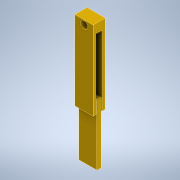
# Autodesk Inventor part: pendel
Saved by Autodesk Inventor 2021 (Build 250183000, 183)
## iProperties
Created: 2021-02-09
Part Number: pendel
Material: Generic
Document SubType Name: Modeling
Designer: Emil
Density: 1 g/cm^3
Appearance: Gold
Author: Emil
Autodesk Inventor part; units mm, degrees
ref_plane "YZ Plane" through (0, 0, 0) normal (1, 0, 0) x (0, 1, 0)
ref_plane "XZ Plane" through (0, 0, 0) normal (0, 1, 0) x (-1, 0, 0)
ref_plane "XY Plane" through (0, 0, 0) normal (0, 0, 1) x (1, 0, 0)
sketch "Sketch1" plane through (0, 0, 0) normal (0, 0, 1) x (1, 0, 0)
  point P0 (0, 0)
sketch "Sketch2" plane through (0, 0, 0) normal (0, 0, 1) x (1, 0, 0)
  line L0 (-15, 130) -> (15, 130)
  line L1 (15, 130) -> (15, 0)
  line L2 (15, 0) -> (-15, 0)
  line L3 (-15, 0) -> (-15, 130)
  point P0 (0, 0)
  point P1 (0, 0)
  dimension "d0" = 30
  dimension "d1" = 130
  constraints: 8 end point, 2 parallel, 1 coincident, 1 horizontal, 1 midpoint, 1 perpendicular
  measures "d0" distance of L0.start L0.end
  measures "d1" distance of L0.end L1.end
extrude "Extrusion1" add sketch "Sketch2" along normal blind 5
ref_plane "Work Plane1" through (0, 0, -10) normal (0, 0, -1) x (-1, 0, 0)
sketch "Sketch4" plane through (0, 0, -10) normal (0, 0, -1) x (-1, 0, 0)
  line L0 (-15, 0) -> (-15, 130) projected
  line L1 (15, 0) -> (-15, 0) projected
  line L2 (-15, 130) -> (15, 130)
  line L3 (15, 130) -> (15, 0)
  line L4 (15, 0) -> (-15, 0)
  line L5 (-15, 0) -> (-15, 130)
  point P0 (0, 0)
  constraints: 8 end point, 2 parallel, 1 horizontal, 1 perpendicular
extrude "Extrusion3" add sketch "Sketch4" along normal blind 5
sketch "Sketch5" plane through (0, 0, -10) normal (0, 0, 1) x (1, 0, 0)
  line L0 (-15, 130) -> (-15, 0) projected
  line L1 (15, 130) -> (15, 0) projected
  line L2 (-15, 130) -> (15, 130)
  line L3 (15, 130) -> (15, 115)
  line L4 (15, 115) -> (-15, 115)
  line L5 (-15, 115) -> (-15, 130)
  point P0 (0, 0)
  point P1 (15, 130)
  dimension "d12" = 15
  constraints: 8 end point, 2 parallel, 1 horizontal, 1 perpendicular, 1 point on line
  measures "d12" distance between parallel lines of L4 L2
extrude "Extrusion4" add sketch "Sketch5" along normal blind 10
sketch "Sketch6" plane through (0, 0, -10) normal (0, 0, 1) x (1, 0, 0)
  circle A0 centre (0, 10) radius 2.5
  line L0 (-15, 0) -> (15, 0) projected
  point P0 (0, 0)
  dimension "d15" = 5
  dimension "d16" = 10
  dimension "d45" = 18.0278
  constraints: 1 centre point
  measures "d15" diameter of A0
  measures "d16" distance from line of L0 A0.centre
  measures "d45" distance of L0.end A0.centre
extrude "Extrusion5" add sketch "Sketch6" along normal blind 10
ref_plane "Work Plane2" through (0, 0, -5) normal (0, 0, 1) x (1, 0, 0)
sketch "Sketch7" plane through (0, 0, -5) normal (0, 0, 1) x (1, 0, 0)
  line L0 (-15, 0) -> (-15, 115) projected
  line L1 (-15, 20) -> (15, 20)
  line L2 (15, 20) -> (15, -80)
  line L3 (15, -80) -> (-15, -80)
  line L4 (-15, -80) -> (-15, 20)
  line L5 (15, 0) -> (-15, 0) projected
  circle A0 centre (0, 10) radius 2.5 projected
  circle A1 centre (0, 10) radius 4
  point P0 (0, 0)
  dimension "d20" = 30
  dimension "d21" = 100
  dimension "d22" = 20
  dimension "d23" = 8
  constraints: 8 end point, 2 parallel, 1 centre point, 1 coincident, 1 horizontal, 1 perpendicular, 1 point on line
  measures "d20" distance between parallel lines of L4 L2
  measures "d21" distance of L1.end L2.end
  measures "d22" distance between parallel lines of L5 L1
  measures "d23" diameter of A1
extrude "Extrusion6" add sketch "Sketch7" along normal mid plane 7 contours L5 L2 L3 L4 | L0 L1 L2 L5
sketch "Sketch9" plane through (0, 0, 5) normal (0, 0, 1) x (1, 0, 0)
  line L0 (15, 130) -> (-15, 130) projected
  line L1 (15, 0) -> (15, 130) projected
  line L2 (0, 84.3715) -> (0, -83.7026)
  line L3 (-15, 0) -> (15, 0) projected
  line L4 (-15, 122.5) -> (15, 122.5)
  line L5 (-15, 115) -> (15, 115) projected
  circle A0 centre (0, 122.5) radius 6
  point P0 (0, 0)
  point P1 (0, 0)
  dimension "d41" = 7.5
  dimension "d42" = 12
  dimension "d46" = 15
  dimension "d47" = 45.6285
  dimension "d48" = 213.7026
  constraints: 4 end point, 2 midpoint, 2 point on line, 1 centre point, 1 perpendicular, 1 vertical
  measures "d41" distance between parallel lines of L5 L4
  measures "d42" diameter of A0
  measures "d46" distance from line of A0.centre L1
  measures "d47" distance from line of L2.start L0
  measures "d48" distance from line of L2.end L0
sketch "Sketch10" plane through (0, 0, -1.5) normal (0, 0, 1) x (1, 0, 0)
  point P0 (0, 0)
sketch "Sketch11" plane through (-15, -80, -1.5) normal (-1, 0, 0) x (0, 0, 1)
  line L0 (-5.6394, 0.8654) -> (-5.6394, 102.3274) construction
  line L1 (-5.6394, 102.3274) -> (-2.3913, 102.3274) construction
  line L2 (-2.3913, 102.3274) -> (-2.3913, 0.8654) construction
  line L3 (-2.3913, 0.8654) -> (-5.6394, 0.8654) construction
  line L4 (-5.6394, 1.7568) -> (-4.0835, 1.6401)
  line L5 (-4.0835, 1.6401) -> (-4.0835, 1.2868)
  line L6 (-4.0835, 1.2868) -> (-5.6394, 1.1701)
  line L7 (-5.6394, 1.1701) -> (-5.6394, 1.7568)
  line L8 (-5.6394, 2.7681) -> (-4.0835, 2.6514)
  line L9 (-4.0835, 2.6514) -> (-4.0835, 2.2981)
  line L10 (-4.0835, 2.2981) -> (-5.6394, 2.1814)
  line L11 (-5.6394, 2.1814) -> (-5.6394, 2.7681)
  line L12 (-1.4611, 4.8719) -> (-1.4611, 3.3224)
  line L13 (-1.4611, 3.3224) -> (-1.8695, 3.3224)
  line L14 (-1.8695, 3.3224) -> (-1.8695, 3.8313)
  line L15 (-1.8695, 3.8313) -> (-5.0527, 3.8313)
  line L16 (-5.0527, 3.8313) -> (-5.0527, 3.3224)
  line L17 (-5.0527, 3.3224) -> (-5.4611, 3.3224)
  line L18 (-5.4611, 3.3224) -> (-5.4611, 4.8719)
  line L19 (-5.4611, 4.8719) -> (-5.0527, 4.8719)
  line L20 (-5.0527, 4.8719) -> (-5.0527, 4.3629)
  line L21 (-5.0527, 4.3629) -> (-1.8695, 4.3629)
  line L22 (-1.8695, 4.3629) -> (-1.8695, 4.8719)
  line L23 (-1.8695, 4.8719) -> (-1.4611, 4.8719)
  spline S0 degree 2 poles (-1.4028, 8.1166) (-1.4028, 7.7049) (-1.8728, 7.2414) (-2.3817, 7.2414) knots 0 0 0 1 2 2 2
  line L24 (-2.3817, 7.2414) -> (-4.0446, 7.2414)
  line L25 (-4.0446, 7.2414) -> (-4.0446, 6.901)
  line L26 (-4.0446, 6.901) -> (-4.4627, 6.901)
  line L27 (-4.4627, 6.901) -> (-4.4627, 7.2414)
  line L28 (-4.4627, 7.2414) -> (-5.325, 7.2414)
  line L29 (-5.325, 7.2414) -> (-5.325, 7.7471)
  line L30 (-5.325, 7.7471) -> (-4.4627, 7.7471)
  line L31 (-4.4627, 7.7471) -> (-4.4627, 8.6774)
  line L32 (-4.4627, 8.6774) -> (-4.0446, 8.6774)
  line L33 (-4.0446, 8.6774) -> (-4.0446, 7.7471)
  line L34 (-4.0446, 7.7471) -> (-2.6151, 7.7471)
  spline S1 degree 2 poles (-2.6151, 7.7471) (-2.3882, 7.7471) (-2.1386, 7.7633) (-2.0316, 7.8184) knots 0 0 0 1 2 2 2
  spline S2 degree 2 poles (-2.0316, 7.8184) (-1.9376, 7.8638) (-1.8436, 8.068) (-1.8436, 8.243) knots 0 0 0 1 2 2 2
  spline S3 degree 2 poles (-1.8436, 8.243) (-1.8436, 8.3662) (-1.9182, 8.5963) (-1.9408, 8.6482) knots 0 0 0 1 2 2 2
  line L35 (-1.9408, 8.6482) -> (-1.9408, 8.6774)
  line L36 (-1.9408, 8.6774) -> (-1.487, 8.6774)
  spline S4 degree 2 poles (-1.487, 8.6774) (-1.4481, 8.5347) (-1.4028, 8.243) (-1.4028, 8.1166) knots 0 0 0 1 2 2 2
  line L37 (-1.4611, 11.4067) -> (-1.4611, 10.901)
  line L38 (-1.4611, 10.901) -> (-3.1726, 10.901)
  spline S5 degree 2 poles (-3.1726, 10.901) (-3.3801, 10.901) (-3.7366, 10.8621) (-3.8436, 10.8038) knots 0 0 0 1 2 2 2
  spline S6 degree 2 poles (-3.8436, 10.8038) (-3.957, 10.7422) (-4.0673, 10.5218) (-4.0673, 10.3338) knots 0 0 0 1 2 2 2
  spline S7 degree 2 poles (-4.0673, 10.3338) (-4.0673, 10.1458) (-3.8663, 9.7471) (-3.7042, 9.5558) knots 0 0 0 1 2 2 2
  line L39 (-3.7042, 9.5558) -> (-1.4611, 9.5558)
  line L40 (-1.4611, 9.5558) -> (-1.4611, 9.0501)
  line L41 (-1.4611, 9.0501) -> (-5.6394, 9.0501)
  line L42 (-5.6394, 9.0501) -> (-5.6394, 9.5558)
  line L43 (-5.6394, 9.5558) -> (-4.1288, 9.5558)
  spline S8 degree 2 poles (-4.1288, 9.5558) (-4.3331, 9.7827) (-4.547, 10.2203) (-4.547, 10.4667) knots 0 0 0 1 2 2 2
  spline S9 degree 2 poles (-4.547, 10.4667) (-4.547, 10.9075) (-3.9635, 11.4067) (-3.4092, 11.4067) knots 0 0 0 1 2 2 2
  line L44 (-3.4092, 11.4067) -> (-1.4611, 11.4067)
  line L45 (-3.9214, 13.7082) -> (-3.9214, 13.6822)
  spline S10 degree 2 poles (-3.9214, 13.6822) (-3.9376, 13.6239) (-3.9441, 13.4975) (-3.9441, 13.4099) knots 0 0 0 1 2 2 2
  spline S11 degree 2 poles (-3.9441, 13.4099) (-3.9441, 13.2057) (-3.7658, 12.8038) (-3.5908, 12.6223) knots 0 0 0 1 2 2 2
  line L46 (-3.5908, 12.6223) -> (-1.4611, 12.6223)
  line L47 (-1.4611, 12.6223) -> (-1.4611, 12.1166)
  line L48 (-1.4611, 12.1166) -> (-4.4627, 12.1166)
  line L49 (-4.4627, 12.1166) -> (-4.4627, 12.6223)
  line L50 (-4.4627, 12.6223) -> (-4.0154, 12.6223)
  spline S12 degree 2 poles (-4.0154, 12.6223) (-4.2618, 12.8978) (-4.4627, 13.3095) (-4.4627, 13.5039) knots 0 0 0 1 2 2 2
  spline S13 degree 2 poles (-4.4627, 13.5039) (-4.4627, 13.5817) (-4.4562, 13.6595) (-4.4465, 13.7082) knots 0 0 0 1 2 2 2
  line L51 (-4.4465, 13.7082) -> (-3.9214, 13.7082)
  line L52 (-1.4611, 14.6158) -> (-1.4611, 14.1101)
  line L53 (-1.4611, 14.1101) -> (-4.4627, 14.1101)
  line L54 (-4.4627, 14.1101) -> (-4.4627, 14.6158)
  line L55 (-4.4627, 14.6158) -> (-1.4611, 14.6158)
  line L56 (-4.9619, 14.6514) -> (-4.9619, 14.0777)
  line L57 (-4.9619, 14.0777) -> (-5.487, 14.0777)
  line L58 (-5.487, 14.0777) -> (-5.487, 14.6514)
  line L59 (-5.487, 14.6514) -> (-4.9619, 14.6514)
  line L60 (-4.4627, 17.7146) -> (-1.4611, 16.5834)
  line L61 (-1.4611, 16.5834) -> (-1.4611, 16.1296)
  line L62 (-1.4611, 16.1296) -> (-4.4627, 15.008)
  line L63 (-4.4627, 15.008) -> (-4.4627, 15.5558)
  line L64 (-4.4627, 15.5558) -> (-2.1515, 16.3759)
  line L65 (-2.1515, 16.3759) -> (-4.4627, 17.1895)
  line L66 (-4.4627, 17.1895) -> (-4.4627, 17.7146)
  spline S14 degree 2 poles (-1.393, 19.4002) (-1.393, 18.6806) (-2.2002, 17.8897) (-2.9457, 17.8897) knots 0 0 0 1 2 2 2
  spline S15 degree 2 poles (-2.9457, 17.8897) (-3.6783, 17.8897) (-4.547, 18.6579) (-4.547, 19.277) knots 0 0 0 1 2 2 2
  spline S16 degree 2 poles (-4.547, 19.277) (-4.547, 19.5558) (-4.3849, 19.9869) (-4.2131, 20.1458) knots 0 0 0 1 2 2 2
  spline S17 degree 2 poles (-4.2131, 20.1458) (-4.0413, 20.3078) (-3.5454, 20.4796) (-3.1856, 20.4796) knots 0 0 0 1 2 2 2
  line L67 (-3.1856, 20.4796) -> (-2.91, 20.4796)
  line L68 (-2.91, 20.4796) -> (-2.91, 18.4018)
  spline S18 degree 2 poles (-2.91, 18.4018) (-2.3882, 18.4018) (-1.8339, 18.927) (-1.8339, 19.3937) knots 0 0 0 1 2 2 2
  spline S19 degree 2 poles (-1.8339, 19.3937) (-1.8339, 19.5591) (-1.9084, 19.88) (-1.9668, 20.0096) knots 0 0 0 1 2 2 2
  spline S20 degree 2 poles (-1.9668, 20.0096) (-2.0316, 20.1458) (-2.1451, 20.3338) (-2.1969, 20.3954) knots 0 0 0 1 2 2 2
  line L69 (-2.1969, 20.3954) -> (-2.1969, 20.4245)
  line L70 (-2.1969, 20.4245) -> (-1.6459, 20.4245)
  spline S21 degree 2 poles (-1.6459, 20.4245) (-1.6102, 20.337) (-1.5065, 20.0712) (-1.4773, 19.9675) knots 0 0 0 1 2 2 2
  spline S22 degree 2 poles (-1.4773, 19.9675) (-1.4352, 19.8216) (-1.393, 19.5817) (-1.393, 19.4002) knots 0 0 0 1 2 2 2
  spline S23 degree 2 poles (-3.2958, 19.9869) (-3.5, 19.9804) (-3.7982, 19.8962) (-3.8987, 19.8151) knots 0 0 0 1 2 2 2
  spline S24 degree 2 poles (-3.8987, 19.8151) (-4.0122, 19.7276) (-4.1321, 19.4521) (-4.1321, 19.2479) knots 0 0 0 1 2 2 2
  spline S25 degree 2 poles (-4.1321, 19.2479) (-4.1321, 19.0469) (-4.0122, 18.7649) (-3.8955, 18.6482) knots 0 0 0 1 2 2 2
  spline S26 degree 2 poles (-3.8955, 18.6482) (-3.7755, 18.5347) (-3.487, 18.418) (-3.2958, 18.4018) knots 0 0 0 1 2 2 2
  line L71 (-3.2958, 18.4018) -> (-3.2958, 19.9869)
  line L72 (-1.4611, 23.2252) -> (-1.4611, 22.7195)
  line L73 (-1.4611, 22.7195) -> (-4.4627, 22.7195)
  line L74 (-4.4627, 22.7195) -> (-4.4627, 23.2252)
  line L75 (-4.4627, 23.2252) -> (-1.4611, 23.2252)
  line L76 (-4.9619, 23.2608) -> (-4.9619, 22.6871)
  line L77 (-4.9619, 22.6871) -> (-5.487, 22.6871)
  line L78 (-5.487, 22.6871) -> (-5.487, 23.2608)
  line L79 (-5.487, 23.2608) -> (-4.9619, 23.2608)
  line L80 (-1.4611, 26.324) -> (-1.4611, 25.8184)
  line L81 (-1.4611, 25.8184) -> (-3.1726, 25.8184)
  spline S27 degree 2 poles (-3.1726, 25.8184) (-3.3801, 25.8184) (-3.7366, 25.7795) (-3.8436, 25.7211) knots 0 0 0 1 2 2 2
  spline S28 degree 2 poles (-3.8436, 25.7211) (-3.957, 25.6595) (-4.0673, 25.4391) (-4.0673, 25.2511) knots 0 0 0 1 2 2 2
  spline S29 degree 2 poles (-4.0673, 25.2511) (-4.0673, 25.0631) (-3.8663, 24.6644) (-3.7042, 24.4732) knots 0 0 0 1 2 2 2
  line L82 (-3.7042, 24.4732) -> (-1.4611, 24.4732)
  line L83 (-1.4611, 24.4732) -> (-1.4611, 23.9675)
  line L84 (-1.4611, 23.9675) -> (-4.4627, 23.9675)
  line L85 (-4.4627, 23.9675) -> (-4.4627, 24.4732)
  line L86 (-4.4627, 24.4732) -> (-4.1288, 24.4732)
  spline S30 degree 2 poles (-4.1288, 24.4732) (-4.3331, 24.7001) (-4.547, 25.1377) (-4.547, 25.384) knots 0 0 0 1 2 2 2
  spline S31 degree 2 poles (-4.547, 25.384) (-4.547, 25.8249) (-3.9635, 26.324) (-3.4092, 26.324) knots 0 0 0 1 2 2 2
  line L87 (-3.4092, 26.324) -> (-1.4611, 26.324)
  spline S32 degree 2 poles (-1.3898, 29.5623) (-1.3898, 29.2608) (-1.5519, 28.739) (-1.6426, 28.5672) knots 0 0 0 1 2 2 2
  line L88 (-1.6426, 28.5672) -> (-2.2099, 28.5672)
  line L89 (-2.2099, 28.5672) -> (-2.2099, 28.5931)
  spline S33 degree 2 poles (-2.2099, 28.5931) (-2.158, 28.6579) (-2.0348, 28.833) (-1.9668, 28.9788) knots 0 0 0 1 2 2 2
  spline S34 degree 2 poles (-1.9668, 28.9788) (-1.9052, 29.1052) (-1.8144, 29.4164) (-1.8144, 29.5817) knots 0 0 0 1 2 2 2
  spline S35 degree 2 poles (-1.8144, 29.5817) (-1.8144, 29.7017) (-1.8695, 29.9772) (-1.9149, 30.042) knots 0 0 0 1 2 2 2
  spline S36 degree 2 poles (-1.9149, 30.042) (-1.9765, 30.136) (-2.1159, 30.2203) (-2.2585, 30.2203) knots 0 0 0 1 2 2 2
  spline S37 degree 2 poles (-2.2585, 30.2203) (-2.4368, 30.2203) (-2.6216, 30.0258) (-2.6831, 29.7762) knots 0 0 0 1 2 2 2
  spline S38 degree 2 poles (-2.6831, 29.7762) (-2.7058, 29.679) (-2.7707, 29.3678) (-2.8063, 29.2349) knots 0 0 0 1 2 2 2
  spline S39 degree 2 poles (-2.8063, 29.2349) (-2.9068, 28.8913) (-3.3217, 28.5801) (-3.6167, 28.5801) knots 0 0 0 1 2 2 2
  spline S40 degree 2 poles (-3.6167, 28.5801) (-4.0251, 28.5801) (-4.534, 29.1928) (-4.534, 29.6984) knots 0 0 0 1 2 2 2
  spline S41 degree 2 poles (-4.534, 29.6984) (-4.534, 29.948) (-4.4109, 30.4537) (-4.3169, 30.6255) knots 0 0 0 1 2 2 2
  line L90 (-4.3169, 30.6255) -> (-3.7755, 30.6255)
  line L91 (-3.7755, 30.6255) -> (-3.7755, 30.5996)
  spline S42 degree 2 poles (-3.7755, 30.5996) (-3.9311, 30.4051) (-4.1094, 29.9318) (-4.1094, 29.6887) knots 0 0 0 1 2 2 2
  spline S43 degree 2 poles (-4.1094, 29.6887) (-4.1094, 29.4391) (-3.8987, 29.0955) (-3.688, 29.0955) knots 0 0 0 1 2 2 2
  spline S44 degree 2 poles (-3.688, 29.0955) (-3.4968, 29.0955) (-3.312, 29.2997) (-3.2536, 29.5266) knots 0 0 0 1 2 2 2
  spline S45 degree 2 poles (-3.2536, 29.5266) (-3.2245, 29.6368) (-3.1661, 29.9156) (-3.1305, 30.068) knots 0 0 0 1 2 2 2
  spline S46 degree 2 poles (-3.1305, 30.068) (-3.0462, 30.3986) (-2.6605, 30.7357) (-2.3266, 30.7357) knots 0 0 0 1 2 2 2
  spline S47 degree 2 poles (-2.3266, 30.7357) (-2.1321, 30.7357) (-1.7885, 30.5834) (-1.6621, 30.4343) knots 0 0 0 1 2 2 2
  spline S48 degree 2 poles (-1.6621, 30.4343) (-1.5292, 30.2754) (-1.3898, 29.8702) (-1.3898, 29.5623) knots 0 0 0 1 2 2 2
  spline S49 degree 2 poles (-1.4028, 32.1133) (-1.4028, 31.7017) (-1.8728, 31.2381) (-2.3817, 31.2381) knots 0 0 0 1 2 2 2
  line L92 (-2.3817, 31.2381) -> (-4.0446, 31.2381)
  line L93 (-4.0446, 31.2381) -> (-4.0446, 30.8978)
  line L94 (-4.0446, 30.8978) -> (-4.4627, 30.8978)
  line L95 (-4.4627, 30.8978) -> (-4.4627, 31.2381)
  line L96 (-4.4627, 31.2381) -> (-5.325, 31.2381)
  line L97 (-5.325, 31.2381) -> (-5.325, 31.7438)
  line L98 (-5.325, 31.7438) -> (-4.4627, 31.7438)
  line L99 (-4.4627, 31.7438) -> (-4.4627, 32.6741)
  line L100 (-4.4627, 32.6741) -> (-4.0446, 32.6741)
  line L101 (-4.0446, 32.6741) -> (-4.0446, 31.7438)
  line L102 (-4.0446, 31.7438) -> (-2.6151, 31.7438)
  spline S50 degree 2 poles (-2.6151, 31.7438) (-2.3882, 31.7438) (-2.1386, 31.76) (-2.0316, 31.8151) knots 0 0 0 1 2 2 2
  spline S51 degree 2 poles (-2.0316, 31.8151) (-1.9376, 31.8605) (-1.8436, 32.0647) (-1.8436, 32.2398) knots 0 0 0 1 2 2 2
  spline S52 degree 2 poles (-1.8436, 32.2398) (-1.8436, 32.3629) (-1.9182, 32.5931) (-1.9408, 32.645) knots 0 0 0 1 2 2 2
  line L103 (-1.9408, 32.645) -> (-1.9408, 32.6741)
  line L104 (-1.9408, 32.6741) -> (-1.487, 32.6741)
  spline S53 degree 2 poles (-1.487, 32.6741) (-1.4481, 32.5315) (-1.4028, 32.2398) (-1.4028, 32.1133) knots 0 0 0 1 2 2 2
  line L105 (-3.9214, 34.6385) -> (-3.9214, 34.6125)
  spline S54 degree 2 poles (-3.9214, 34.6125) (-3.9376, 34.5542) (-3.9441, 34.4278) (-3.9441, 34.3403) knots 0 0 0 1 2 2 2
  spline S55 degree 2 poles (-3.9441, 34.3403) (-3.9441, 34.136) (-3.7658, 33.7341) (-3.5908, 33.5526) knots 0 0 0 1 2 2 2
  line L106 (-3.5908, 33.5526) -> (-1.4611, 33.5526)
  line L107 (-1.4611, 33.5526) -> (-1.4611, 33.0469)
  line L108 (-1.4611, 33.0469) -> (-4.4627, 33.0469)
  line L109 (-4.4627, 33.0469) -> (-4.4627, 33.5526)
  line L110 (-4.4627, 33.5526) -> (-4.0154, 33.5526)
  spline S56 degree 2 poles (-4.0154, 33.5526) (-4.2618, 33.8281) (-4.4627, 34.2398) (-4.4627, 34.4343) knots 0 0 0 1 2 2 2
  spline S57 degree 2 poles (-4.4627, 34.4343) (-4.4627, 34.5121) (-4.4562, 34.5898) (-4.4465, 34.6385) knots 0 0 0 1 2 2 2
  line L111 (-4.4465, 34.6385) -> (-3.9214, 34.6385)
  line L112 (-1.4611, 37.3646) -> (-1.4611, 36.8589)
  line L113 (-1.4611, 36.8589) -> (-1.7917, 36.8589)
  spline S58 degree 2 poles (-1.7917, 36.8589) (-1.5875, 36.6255) (-1.3768, 36.2074) (-1.3768, 35.948) knots 0 0 0 1 2 2 2
  spline S59 degree 2 poles (-1.3768, 35.948) (-1.3768, 35.7535) (-1.5065, 35.4067) (-1.6459, 35.2803) knots 0 0 0 1 2 2 2
  spline S60 degree 2 poles (-1.6459, 35.2803) (-1.7853, 35.1506) (-2.2099, 35.008) (-2.5146, 35.008) knots 0 0 0 1 2 2 2
  line L114 (-2.5146, 35.008) -> (-4.4627, 35.008)
  line L115 (-4.4627, 35.008) -> (-4.4627, 35.5137)
  line L116 (-4.4627, 35.5137) -> (-2.7512, 35.5137)
  spline S61 degree 2 poles (-2.7512, 35.5137) (-2.5113, 35.5137) (-2.1969, 35.5493) (-2.0802, 35.6109) knots 0 0 0 1 2 2 2
  spline S62 degree 2 poles (-2.0802, 35.6109) (-1.9635, 35.6725) (-1.8566, 35.8832) (-1.8566, 36.0809) knots 0 0 0 1 2 2 2
  spline S63 degree 2 poles (-1.8566, 36.0809) (-1.8566, 36.2657) (-2.0673, 36.6839) (-2.2196, 36.8589) knots 0 0 0 1 2 2 2
  line L117 (-2.2196, 36.8589) -> (-4.4627, 36.8589)
  line L118 (-4.4627, 36.8589) -> (-4.4627, 37.3646)
  line L119 (-4.4627, 37.3646) -> (-1.4611, 37.3646)
  spline S64 degree 2 poles (-1.393, 39.29) (-1.393, 38.9788) (-1.5843, 38.4634) (-1.7788, 38.2787) knots 0 0 0 1 2 2 2
  spline S65 degree 2 poles (-1.7788, 38.2787) (-1.97, 38.0939) (-2.56, 37.8897) (-2.9554, 37.8897) knots 0 0 0 1 2 2 2
  spline S66 degree 2 poles (-2.9554, 37.8897) (-3.3509, 37.8897) (-3.9279, 38.1004) (-4.1224, 38.2787) knots 0 0 0 1 2 2 2
  spline S67 degree 2 poles (-4.1224, 38.2787) (-4.3201, 38.4569) (-4.5308, 38.9853) (-4.5308, 39.29) knots 0 0 0 1 2 2 2
  spline S68 degree 2 poles (-4.5308, 39.29) (-4.5308, 39.5364) (-4.3914, 39.9967) (-4.3006, 40.1749) knots 0 0 0 1 2 2 2
  line L120 (-4.3006, 40.1749) -> (-3.7334, 40.1749)
  line L121 (-3.7334, 40.1749) -> (-3.7334, 40.1458)
  spline S69 degree 2 poles (-3.7334, 40.1458) (-3.7788, 40.0907) (-3.8955, 39.9221) (-3.957, 39.8022) knots 0 0 0 1 2 2 2
  spline S70 degree 2 poles (-3.957, 39.8022) (-4.0089, 39.6952) (-4.09, 39.4099) (-4.09, 39.2803) knots 0 0 0 1 2 2 2
  spline S71 degree 2 poles (-4.09, 39.2803) (-4.09, 38.8881) (-3.4968, 38.4116) (-2.9554, 38.4116) knots 0 0 0 1 2 2 2
  spline S72 degree 2 poles (-2.9554, 38.4116) (-2.4271, 38.4116) (-1.8339, 38.8719) (-1.8339, 39.2803) knots 0 0 0 1 2 2 2
  spline S73 degree 2 poles (-1.8339, 39.2803) (-1.8339, 39.5266) (-2.0381, 39.974) (-2.1969, 40.1458) knots 0 0 0 1 2 2 2
  line L122 (-2.1969, 40.1458) -> (-2.1969, 40.1749)
  line L123 (-2.1969, 40.1749) -> (-1.6297, 40.1749)
  spline S74 degree 2 poles (-1.6297, 40.1749) (-1.594, 40.1004) (-1.4935, 39.8735) (-1.4708, 39.7827) knots 0 0 0 1 2 2 2
  spline S75 degree 2 poles (-1.4708, 39.7827) (-1.4319, 39.6531) (-1.393, 39.4488) (-1.393, 39.29) knots 0 0 0 1 2 2 2
  spline S76 degree 2 poles (-1.4028, 41.5428) (-1.4028, 41.1312) (-1.8728, 40.6676) (-2.3817, 40.6676) knots 0 0 0 1 2 2 2
  line L124 (-2.3817, 40.6676) -> (-4.0446, 40.6676)
  line L125 (-4.0446, 40.6676) -> (-4.0446, 40.3273)
  line L126 (-4.0446, 40.3273) -> (-4.4627, 40.3273)
  line L127 (-4.4627, 40.3273) -> (-4.4627, 40.6676)
  line L128 (-4.4627, 40.6676) -> (-5.325, 40.6676)
  line L129 (-5.325, 40.6676) -> (-5.325, 41.1733)
  line L130 (-5.325, 41.1733) -> (-4.4627, 41.1733)
  line L131 (-4.4627, 41.1733) -> (-4.4627, 42.1036)
  line L132 (-4.4627, 42.1036) -> (-4.0446, 42.1036)
  line L133 (-4.0446, 42.1036) -> (-4.0446, 41.1733)
  line L134 (-4.0446, 41.1733) -> (-2.6151, 41.1733)
  spline S77 degree 2 poles (-2.6151, 41.1733) (-2.3882, 41.1733) (-2.1386, 41.1895) (-2.0316, 41.2446) knots 0 0 0 1 2 2 2
  spline S78 degree 2 poles (-2.0316, 41.2446) (-1.9376, 41.29) (-1.8436, 41.4942) (-1.8436, 41.6693) knots 0 0 0 1 2 2 2
  spline S79 degree 2 poles (-1.8436, 41.6693) (-1.8436, 41.7924) (-1.9182, 42.0226) (-1.9408, 42.0745) knots 0 0 0 1 2 2 2
  line L135 (-1.9408, 42.0745) -> (-1.9408, 42.1036)
  line L136 (-1.9408, 42.1036) -> (-1.487, 42.1036)
  spline S80 degree 2 poles (-1.487, 42.1036) (-1.4481, 41.961) (-1.4028, 41.6693) (-1.4028, 41.5428) knots 0 0 0 1 2 2 2
  line L137 (-1.4611, 44.8103) -> (-1.4611, 44.3046)
  line L138 (-1.4611, 44.3046) -> (-1.7917, 44.3046)
  spline S81 degree 2 poles (-1.7917, 44.3046) (-1.5875, 44.0712) (-1.3768, 43.6531) (-1.3768, 43.3937) knots 0 0 0 1 2 2 2
  spline S82 degree 2 poles (-1.3768, 43.3937) (-1.3768, 43.1992) (-1.5065, 42.8524) (-1.6459, 42.726) knots 0 0 0 1 2 2 2
  spline S83 degree 2 poles (-1.6459, 42.726) (-1.7853, 42.5963) (-2.2099, 42.4537) (-2.5146, 42.4537) knots 0 0 0 1 2 2 2
  line L139 (-2.5146, 42.4537) -> (-4.4627, 42.4537)
  line L140 (-4.4627, 42.4537) -> (-4.4627, 42.9594)
  line L141 (-4.4627, 42.9594) -> (-2.7512, 42.9594)
  spline S84 degree 2 poles (-2.7512, 42.9594) (-2.5113, 42.9594) (-2.1969, 42.995) (-2.0802, 43.0566) knots 0 0 0 1 2 2 2
  spline S85 degree 2 poles (-2.0802, 43.0566) (-1.9635, 43.1182) (-1.8566, 43.3289) (-1.8566, 43.5266) knots 0 0 0 1 2 2 2
  spline S86 degree 2 poles (-1.8566, 43.5266) (-1.8566, 43.7114) (-2.0673, 44.1296) (-2.2196, 44.3046) knots 0 0 0 1 2 2 2
  line L142 (-2.2196, 44.3046) -> (-4.4627, 44.3046)
  line L143 (-4.4627, 44.3046) -> (-4.4627, 44.8103)
  line L144 (-4.4627, 44.8103) -> (-1.4611, 44.8103)
  line L145 (-3.9214, 47.1344) -> (-3.9214, 47.1085)
  spline S87 degree 2 poles (-3.9214, 47.1085) (-3.9376, 47.0501) (-3.9441, 46.9237) (-3.9441, 46.8362) knots 0 0 0 1 2 2 2
  spline S88 degree 2 poles (-3.9441, 46.8362) (-3.9441, 46.632) (-3.7658, 46.23) (-3.5908, 46.0485) knots 0 0 0 1 2 2 2
  line L146 (-3.5908, 46.0485) -> (-1.4611, 46.0485)
  line L147 (-1.4611, 46.0485) -> (-1.4611, 45.5428)
  line L148 (-1.4611, 45.5428) -> (-4.4627, 45.5428)
  line L149 (-4.4627, 45.5428) -> (-4.4627, 46.0485)
  line L150 (-4.4627, 46.0485) -> (-4.0154, 46.0485)
  spline S89 degree 2 poles (-4.0154, 46.0485) (-4.2618, 46.324) (-4.4627, 46.7357) (-4.4627, 46.9302) knots 0 0 0 1 2 2 2
  spline S90 degree 2 poles (-4.4627, 46.9302) (-4.4627, 47.008) (-4.4562, 47.0858) (-4.4465, 47.1344) knots 0 0 0 1 2 2 2
  line L151 (-4.4465, 47.1344) -> (-3.9214, 47.1344)
  spline S91 degree 2 poles (-1.393, 48.8297) (-1.393, 48.1101) (-2.2002, 47.3192) (-2.9457, 47.3192) knots 0 0 0 1 2 2 2
  spline S92 degree 2 poles (-2.9457, 47.3192) (-3.6783, 47.3192) (-4.547, 48.0874) (-4.547, 48.7065) knots 0 0 0 1 2 2 2
  spline S93 degree 2 poles (-4.547, 48.7065) (-4.547, 48.9853) (-4.3849, 49.4164) (-4.2131, 49.5753) knots 0 0 0 1 2 2 2
  spline S94 degree 2 poles (-4.2131, 49.5753) (-4.0413, 49.7373) (-3.5454, 49.9091) (-3.1856, 49.9091) knots 0 0 0 1 2 2 2
  line L152 (-3.1856, 49.9091) -> (-2.91, 49.9091)
  line L153 (-2.91, 49.9091) -> (-2.91, 47.8313)
  spline S95 degree 2 poles (-2.91, 47.8313) (-2.3882, 47.8313) (-1.8339, 48.3565) (-1.8339, 48.8232) knots 0 0 0 1 2 2 2
  spline S96 degree 2 poles (-1.8339, 48.8232) (-1.8339, 48.9886) (-1.9084, 49.3095) (-1.9668, 49.4391) knots 0 0 0 1 2 2 2
  spline S97 degree 2 poles (-1.9668, 49.4391) (-2.0316, 49.5753) (-2.1451, 49.7633) (-2.1969, 49.8249) knots 0 0 0 1 2 2 2
  line L154 (-2.1969, 49.8249) -> (-2.1969, 49.854)
  line L155 (-2.1969, 49.854) -> (-1.6459, 49.854)
  spline S98 degree 2 poles (-1.6459, 49.854) (-1.6102, 49.7665) (-1.5065, 49.5007) (-1.4773, 49.397) knots 0 0 0 1 2 2 2
  spline S99 degree 2 poles (-1.4773, 49.397) (-1.4352, 49.2511) (-1.393, 49.0112) (-1.393, 48.8297) knots 0 0 0 1 2 2 2
  spline S100 degree 2 poles (-3.2958, 49.4164) (-3.5, 49.4099) (-3.7982, 49.3257) (-3.8987, 49.2446) knots 0 0 0 1 2 2 2
  spline S101 degree 2 poles (-3.8987, 49.2446) (-4.0122, 49.1571) (-4.1321, 48.8816) (-4.1321, 48.6774) knots 0 0 0 1 2 2 2
  spline S102 degree 2 poles (-4.1321, 48.6774) (-4.1321, 48.4764) (-4.0122, 48.1944) (-3.8955, 48.0777) knots 0 0 0 1 2 2 2
  spline S103 degree 2 poles (-3.8955, 48.0777) (-3.7755, 47.9642) (-3.487, 47.8475) (-3.2958, 47.8313) knots 0 0 0 1 2 2 2
  line L156 (-3.2958, 47.8313) -> (-3.2958, 49.4164)
  line L157 (-1.4611, 51.2057) -> (-1.4611, 50.5639)
  line L158 (-1.4611, 50.5639) -> (-2.2261, 50.5639)
  line L159 (-2.2261, 50.5639) -> (-2.2261, 51.2057)
  line L160 (-2.2261, 51.2057) -> (-1.4611, 51.2057)
  line L161 (-1.4611, 55.2381) -> (-1.4611, 53.6887)
  line L162 (-1.4611, 53.6887) -> (-1.8695, 53.6887)
  line L163 (-1.8695, 53.6887) -> (-1.8695, 54.1976)
  line L164 (-1.8695, 54.1976) -> (-5.0527, 54.1976)
  line L165 (-5.0527, 54.1976) -> (-5.0527, 53.6887)
  line L166 (-5.0527, 53.6887) -> (-5.4611, 53.6887)
  line L167 (-5.4611, 53.6887) -> (-5.4611, 55.2381)
  line L168 (-5.4611, 55.2381) -> (-5.0527, 55.2381)
  line L169 (-5.0527, 55.2381) -> (-5.0527, 54.7292)
  line L170 (-5.0527, 54.7292) -> (-1.8695, 54.7292)
  line L171 (-1.8695, 54.7292) -> (-1.8695, 55.2381)
  line L172 (-1.8695, 55.2381) -> (-1.4611, 55.2381)
  line L173 (-1.4611, 59.8832) -> (-1.4611, 59.3775)
  line L174 (-1.4611, 59.3775) -> (-1.7658, 59.3775)
  spline S104 degree 2 poles (-1.7658, 59.3775) (-1.6686, 59.2608) (-1.5389, 59.089) (-1.4838, 58.9723) knots 0 0 0 1 2 2 2
  spline S105 degree 2 poles (-1.4838, 58.9723) (-1.4319, 58.8654) (-1.3768, 58.6352) (-1.3768, 58.4829) knots 0 0 0 1 2 2 2
  spline S106 degree 2 poles (-1.3768, 58.4829) (-1.3768, 58.2365) (-1.581, 57.8216) (-1.7788, 57.6757) knots 0 0 0 1 2 2 2
  spline S107 degree 2 poles (-1.7788, 57.6757) (-1.9765, 57.5299) (-2.56, 57.3678) (-2.9392, 57.3678) knots 0 0 0 1 2 2 2
  spline S108 degree 2 poles (-2.9392, 57.3678) (-3.3347, 57.3678) (-3.9117, 57.572) (-4.1288, 57.7503) knots 0 0 0 1 2 2 2
  spline S109 degree 2 poles (-4.1288, 57.7503) (-4.3233, 57.9156) (-4.547, 58.3792) (-4.547, 58.6352) knots 0 0 0 1 2 2 2
  spline S110 degree 2 poles (-4.547, 58.6352) (-4.547, 58.8589) (-4.4465, 59.1928) (-4.3428, 59.3775) knots 0 0 0 1 2 2 2
  line L175 (-4.3428, 59.3775) -> (-5.6394, 59.3775)
  line L176 (-5.6394, 59.3775) -> (-5.6394, 59.8832)
  line L177 (-5.6394, 59.8832) -> (-1.4611, 59.8832)
  line L178 (-2.1904, 59.3775) -> (-3.9246, 59.3775)
  spline S111 degree 2 poles (-3.9246, 59.3775) (-4.0154, 59.1895) (-4.0835, 58.8913) (-4.0835, 58.7195) knots 0 0 0 1 2 2 2
  spline S112 degree 2 poles (-4.0835, 58.7195) (-4.0835, 58.3305) (-3.5, 57.8897) (-2.9489, 57.8897) knots 0 0 0 1 2 2 2
  spline S113 degree 2 poles (-2.9489, 57.8897) (-2.4173, 57.8897) (-1.8566, 58.2268) (-1.8566, 58.5996) knots 0 0 0 1 2 2 2
  spline S114 degree 2 poles (-1.8566, 58.5996) (-1.8566, 58.7973) (-2.0381, 59.1992) (-2.1904, 59.3775) knots 0 0 0 1 2 2 2
  line L179 (-3.9214, 62.2074) -> (-3.9214, 62.1814)
  spline S115 degree 2 poles (-3.9214, 62.1814) (-3.9376, 62.1231) (-3.9441, 61.9967) (-3.9441, 61.9091) knots 0 0 0 1 2 2 2
  spline S116 degree 2 poles (-3.9441, 61.9091) (-3.9441, 61.7049) (-3.7658, 61.303) (-3.5908, 61.1215) knots 0 0 0 1 2 2 2
  line L180 (-3.5908, 61.1215) -> (-1.4611, 61.1215)
  line L181 (-1.4611, 61.1215) -> (-1.4611, 60.6158)
  line L182 (-1.4611, 60.6158) -> (-4.4627, 60.6158)
  line L183 (-4.4627, 60.6158) -> (-4.4627, 61.1215)
  line L184 (-4.4627, 61.1215) -> (-4.0154, 61.1215)
  spline S117 degree 2 poles (-4.0154, 61.1215) (-4.2618, 61.397) (-4.4627, 61.8086) (-4.4627, 62.0031) knots 0 0 0 1 2 2 2
  spline S118 degree 2 poles (-4.4627, 62.0031) (-4.4627, 62.0809) (-4.4562, 62.1587) (-4.4465, 62.2074) knots 0 0 0 1 2 2 2
  line L185 (-4.4465, 62.2074) -> (-3.9214, 62.2074)
  spline S119 degree 2 poles (-2.9619, 65.0663) (-2.2034, 65.0663) (-1.3768, 64.337) (-1.3768, 63.7276) knots 0 0 0 1 2 2 2
  spline S120 degree 2 poles (-1.3768, 63.7276) (-1.3768, 63.102) (-2.2293, 62.3856) (-2.9619, 62.3856) knots 0 0 0 1 2 2 2
  spline S121 degree 2 poles (-2.9619, 62.3856) (-3.7139, 62.3856) (-4.547, 63.1247) (-4.547, 63.7276) knots 0 0 0 1 2 2 2
  spline S122 degree 2 poles (-4.547, 63.7276) (-4.547, 64.337) (-3.7172, 65.0663) (-2.9619, 65.0663) knots 0 0 0 1 2 2 2
  spline S123 degree 2 poles (-2.9619, 64.5445) (-3.5454, 64.5445) (-4.1126, 64.1198) (-4.1126, 63.7276) knots 0 0 0 1 2 2 2
  spline S124 degree 2 poles (-4.1126, 63.7276) (-4.1126, 63.3354) (-3.5454, 62.9075) (-2.9619, 62.9075) knots 0 0 0 1 2 2 2
  spline S125 degree 2 poles (-2.9619, 62.9075) (-2.3947, 62.9075) (-1.8112, 63.3354) (-1.8112, 63.7276) knots 0 0 0 1 2 2 2
  spline S126 degree 2 poles (-1.8112, 63.7276) (-1.8112, 64.1166) (-2.3849, 64.5445) (-2.9619, 64.5445) knots 0 0 0 1 2 2 2
  line L186 (-4.4627, 69.2219) -> (-1.4611, 68.4602)
  line L187 (-1.4611, 68.4602) -> (-1.4611, 67.9934)
  line L188 (-1.4611, 67.9934) -> (-3.7755, 67.2608)
  line L189 (-3.7755, 67.2608) -> (-1.4611, 66.5315)
  line L190 (-1.4611, 66.5315) -> (-1.4611, 66.068)
  line L191 (-1.4611, 66.068) -> (-4.4627, 65.2997)
  line L192 (-4.4627, 65.2997) -> (-4.4627, 65.8249)
  line L193 (-4.4627, 65.8249) -> (-2.1386, 66.3565)
  line L194 (-2.1386, 66.3565) -> (-4.4627, 67.0663)
  line L195 (-4.4627, 67.0663) -> (-4.4627, 67.4845)
  line L196 (-4.4627, 67.4845) -> (-2.1386, 68.2138)
  line L197 (-2.1386, 68.2138) -> (-4.4627, 68.713)
  line L198 (-4.4627, 68.713) -> (-4.4627, 69.2219)
  line L199 (-1.4611, 72.0226) -> (-1.4611, 71.5169)
  line L200 (-1.4611, 71.5169) -> (-3.1726, 71.5169)
  spline S127 degree 2 poles (-3.1726, 71.5169) (-3.3801, 71.5169) (-3.7366, 71.478) (-3.8436, 71.4197) knots 0 0 0 1 2 2 2
  spline S128 degree 2 poles (-3.8436, 71.4197) (-3.957, 71.3581) (-4.0673, 71.1377) (-4.0673, 70.9497) knots 0 0 0 1 2 2 2
  spline S129 degree 2 poles (-4.0673, 70.9497) (-4.0673, 70.7616) (-3.8663, 70.3629) (-3.7042, 70.1717) knots 0 0 0 1 2 2 2
  line L201 (-3.7042, 70.1717) -> (-1.4611, 70.1717)
  line L202 (-1.4611, 70.1717) -> (-1.4611, 69.666)
  line L203 (-1.4611, 69.666) -> (-4.4627, 69.666)
  line L204 (-4.4627, 69.666) -> (-4.4627, 70.1717)
  line L205 (-4.4627, 70.1717) -> (-4.1288, 70.1717)
  spline S130 degree 2 poles (-4.1288, 70.1717) (-4.3331, 70.3986) (-4.547, 70.8362) (-4.547, 71.0826) knots 0 0 0 1 2 2 2
  spline S131 degree 2 poles (-4.547, 71.0826) (-4.547, 71.5234) (-3.9635, 72.0226) (-3.4092, 72.0226) knots 0 0 0 1 2 2 2
  line L206 (-3.4092, 72.0226) -> (-1.4611, 72.0226)
  line L207 (-1.4611, 74.9659) -> (-1.4611, 74.4602)
  line L208 (-1.4611, 74.4602) -> (-4.4627, 74.4602)
  line L209 (-4.4627, 74.4602) -> (-4.4627, 74.9659)
  line L210 (-4.4627, 74.9659) -> (-1.4611, 74.9659)
  line L211 (-4.9619, 75.0015) -> (-4.9619, 74.4278)
  line L212 (-4.9619, 74.4278) -> (-5.487, 74.4278)
  line L213 (-5.487, 74.4278) -> (-5.487, 75.0015)
  line L214 (-5.487, 75.0015) -> (-4.9619, 75.0015)
  line L215 (-1.4611, 78.0647) -> (-1.4611, 77.5591)
  line L216 (-1.4611, 77.5591) -> (-3.1726, 77.5591)
  spline S132 degree 2 poles (-3.1726, 77.5591) (-3.3801, 77.5591) (-3.7366, 77.5202) (-3.8436, 77.4618) knots 0 0 0 1 2 2 2
  spline S133 degree 2 poles (-3.8436, 77.4618) (-3.957, 77.4002) (-4.0673, 77.1798) (-4.0673, 76.9918) knots 0 0 0 1 2 2 2
  spline S134 degree 2 poles (-4.0673, 76.9918) (-4.0673, 76.8038) (-3.8663, 76.4051) (-3.7042, 76.2138) knots 0 0 0 1 2 2 2
  line L217 (-3.7042, 76.2138) -> (-1.4611, 76.2138)
  line L218 (-1.4611, 76.2138) -> (-1.4611, 75.7082)
  line L219 (-1.4611, 75.7082) -> (-4.4627, 75.7082)
  line L220 (-4.4627, 75.7082) -> (-4.4627, 76.2138)
  line L221 (-4.4627, 76.2138) -> (-4.1288, 76.2138)
  spline S135 degree 2 poles (-4.1288, 76.2138) (-4.3331, 76.4407) (-4.547, 76.8783) (-4.547, 77.1247) knots 0 0 0 1 2 2 2
  spline S136 degree 2 poles (-4.547, 77.1247) (-4.547, 77.5655) (-3.9635, 78.0647) (-3.4092, 78.0647) knots 0 0 0 1 2 2 2
  line L222 (-3.4092, 78.0647) -> (-1.4611, 78.0647)
  spline S137 degree 2 poles (-1.393, 81.6855) (-1.393, 81.3743) (-1.5843, 80.8589) (-1.7788, 80.6741) knots 0 0 0 1 2 2 2
  spline S138 degree 2 poles (-1.7788, 80.6741) (-1.97, 80.4894) (-2.56, 80.2851) (-2.9554, 80.2851) knots 0 0 0 1 2 2 2
  spline S139 degree 2 poles (-2.9554, 80.2851) (-3.3509, 80.2851) (-3.9279, 80.4958) (-4.1224, 80.6741) knots 0 0 0 1 2 2 2
  spline S140 degree 2 poles (-4.1224, 80.6741) (-4.3201, 80.8524) (-4.5308, 81.3808) (-4.5308, 81.6855) knots 0 0 0 1 2 2 2
  spline S141 degree 2 poles (-4.5308, 81.6855) (-4.5308, 81.9318) (-4.3914, 82.3921) (-4.3006, 82.5704) knots 0 0 0 1 2 2 2
  line L223 (-4.3006, 82.5704) -> (-3.7334, 82.5704)
  line L224 (-3.7334, 82.5704) -> (-3.7334, 82.5412)
  spline S142 degree 2 poles (-3.7334, 82.5412) (-3.7788, 82.4861) (-3.8955, 82.3176) (-3.957, 82.1976) knots 0 0 0 1 2 2 2
  spline S143 degree 2 poles (-3.957, 82.1976) (-4.0089, 82.0907) (-4.09, 81.8054) (-4.09, 81.6757) knots 0 0 0 1 2 2 2
  spline S144 degree 2 poles (-4.09, 81.6757) (-4.09, 81.2835) (-3.4968, 80.807) (-2.9554, 80.807) knots 0 0 0 1 2 2 2
  spline S145 degree 2 poles (-2.9554, 80.807) (-2.4271, 80.807) (-1.8339, 81.2673) (-1.8339, 81.6757) knots 0 0 0 1 2 2 2
  spline S146 degree 2 poles (-1.8339, 81.6757) (-1.8339, 81.9221) (-2.0381, 82.3694) (-2.1969, 82.5412) knots 0 0 0 1 2 2 2
  line L225 (-2.1969, 82.5412) -> (-2.1969, 82.5704)
  line L226 (-2.1969, 82.5704) -> (-1.6297, 82.5704)
  spline S147 degree 2 poles (-1.6297, 82.5704) (-1.594, 82.4958) (-1.4935, 82.2689) (-1.4708, 82.1782) knots 0 0 0 1 2 2 2
  spline S148 degree 2 poles (-1.4708, 82.1782) (-1.4319, 82.0485) (-1.393, 81.8443) (-1.393, 81.6855) knots 0 0 0 1 2 2 2
  line L227 (-1.4611, 85.3873) -> (-1.4611, 84.8816)
  line L228 (-1.4611, 84.8816) -> (-3.1726, 84.8816)
  spline S149 degree 2 poles (-3.1726, 84.8816) (-3.3801, 84.8816) (-3.7366, 84.8427) (-3.8436, 84.7843) knots 0 0 0 1 2 2 2
  spline S150 degree 2 poles (-3.8436, 84.7843) (-3.957, 84.7227) (-4.0673, 84.5023) (-4.0673, 84.3143) knots 0 0 0 1 2 2 2
  spline S151 degree 2 poles (-4.0673, 84.3143) (-4.0673, 84.1263) (-3.8663, 83.7276) (-3.7042, 83.5364) knots 0 0 0 1 2 2 2
  line L229 (-3.7042, 83.5364) -> (-1.4611, 83.5364)
  line L230 (-1.4611, 83.5364) -> (-1.4611, 83.0307)
  line L231 (-1.4611, 83.0307) -> (-5.6394, 83.0307)
  line L232 (-5.6394, 83.0307) -> (-5.6394, 83.5364)
  line L233 (-5.6394, 83.5364) -> (-4.1288, 83.5364)
  spline S152 degree 2 poles (-4.1288, 83.5364) (-4.3331, 83.7633) (-4.547, 84.2009) (-4.547, 84.4472) knots 0 0 0 1 2 2 2
  spline S153 degree 2 poles (-4.547, 84.4472) (-4.547, 84.8881) (-3.9635, 85.3873) (-3.4092, 85.3873) knots 0 0 0 1 2 2 2
  line L234 (-3.4092, 85.3873) -> (-1.4611, 85.3873)
  spline S154 degree 2 poles (-1.7788, 87.7698) (-1.7334, 87.7082) (-1.5713, 87.5007) (-1.5227, 87.4035) knots 0 0 0 1 2 2 2
  spline S155 degree 2 poles (-1.5227, 87.4035) (-1.4514, 87.2706) (-1.3768, 87.021) (-1.3768, 86.7941) knots 0 0 0 1 2 2 2
  spline S156 degree 2 poles (-1.3768, 86.7941) (-1.3768, 86.6093) (-1.5162, 86.2754) (-1.6426, 86.149) knots 0 0 0 1 2 2 2
  spline S157 degree 2 poles (-1.6426, 86.149) (-1.7658, 86.0291) (-2.1288, 85.8832) (-2.3298, 85.8832) knots 0 0 0 1 2 2 2
  spline S158 degree 2 poles (-2.3298, 85.8832) (-2.641, 85.8832) (-3.0818, 86.1458) (-3.2083, 86.431) knots 0 0 0 1 2 2 2
  spline S159 degree 2 poles (-3.2083, 86.431) (-3.325, 86.6839) (-3.4125, 87.371) (-3.4352, 87.7698) knots 0 0 0 1 2 2 2
  line L235 (-3.4352, 87.7698) -> (-3.5324, 87.7698)
  spline S160 degree 2 poles (-3.5324, 87.7698) (-3.7075, 87.7698) (-3.9246, 87.6628) (-3.9862, 87.5655) knots 0 0 0 1 2 2 2
  spline S161 degree 2 poles (-3.9862, 87.5655) (-4.0478, 87.4683) (-4.0867, 87.1895) (-4.0867, 87.0404) knots 0 0 0 1 2 2 2
  spline S162 degree 2 poles (-4.0867, 87.0404) (-4.0867, 86.8654) (-3.983, 86.3921) (-3.8825, 86.1555) knots 0 0 0 1 2 2 2
  line L236 (-3.8825, 86.1555) -> (-3.8825, 86.1263)
  line L237 (-3.8825, 86.1263) -> (-4.3979, 86.1263)
  spline S163 degree 2 poles (-4.3979, 86.1263) (-4.4368, 86.2657) (-4.534, 86.7876) (-4.534, 87.0437) knots 0 0 0 1 2 2 2
  spline S164 degree 2 poles (-4.534, 87.0437) (-4.534, 87.3548) (-4.4368, 87.7795) (-4.3104, 87.948) knots 0 0 0 1 2 2 2
  spline S165 degree 2 poles (-4.3104, 87.948) (-4.1872, 88.1133) (-3.795, 88.2754) (-3.513, 88.2754) knots 0 0 0 1 2 2 2
  line L238 (-3.513, 88.2754) -> (-1.4611, 88.2754)
  line L239 (-1.4611, 88.2754) -> (-1.4611, 87.7698)
  line L240 (-1.4611, 87.7698) -> (-1.7788, 87.7698)
  line L241 (-2.2002, 87.7698) -> (-3.0332, 87.7698)
  spline S166 degree 2 poles (-3.0332, 87.7698) (-3.017, 87.5882) (-2.9619, 87.0404) (-2.91, 86.8686) knots 0 0 0 1 2 2 2
  spline S167 degree 2 poles (-2.91, 86.8686) (-2.8485, 86.6676) (-2.5924, 86.4051) (-2.3655, 86.4051) knots 0 0 0 1 2 2 2
  spline S168 degree 2 poles (-2.3655, 86.4051) (-2.1062, 86.4051) (-1.8436, 86.6968) (-1.8436, 86.9756) knots 0 0 0 1 2 2 2
  spline S169 degree 2 poles (-1.8436, 86.9756) (-1.8436, 87.2122) (-2.0478, 87.6012) (-2.2002, 87.7698) knots 0 0 0 1 2 2 2
  spline S170 degree 2 poles (-2.9619, 91.4521) (-2.2034, 91.4521) (-1.3768, 90.7227) (-1.3768, 90.1133) knots 0 0 0 1 2 2 2
  spline S171 degree 2 poles (-1.3768, 90.1133) (-1.3768, 89.4877) (-2.2293, 88.7714) (-2.9619, 88.7714) knots 0 0 0 1 2 2 2
  spline S172 degree 2 poles (-2.9619, 88.7714) (-3.7139, 88.7714) (-4.547, 89.5104) (-4.547, 90.1133) knots 0 0 0 1 2 2 2
  spline S173 degree 2 poles (-4.547, 90.1133) (-4.547, 90.7227) (-3.7172, 91.4521) (-2.9619, 91.4521) knots 0 0 0 1 2 2 2
  spline S174 degree 2 poles (-2.9619, 90.9302) (-3.5454, 90.9302) (-4.1126, 90.5056) (-4.1126, 90.1133) knots 0 0 0 1 2 2 2
  spline S175 degree 2 poles (-4.1126, 90.1133) (-4.1126, 89.7211) (-3.5454, 89.2933) (-2.9619, 89.2933) knots 0 0 0 1 2 2 2
  spline S176 degree 2 poles (-2.9619, 89.2933) (-2.3947, 89.2933) (-1.8112, 89.7211) (-1.8112, 90.1133) knots 0 0 0 1 2 2 2
  spline S177 degree 2 poles (-1.8112, 90.1133) (-1.8112, 90.5023) (-2.3849, 90.9302) (-2.9619, 90.9302) knots 0 0 0 1 2 2 2
  spline S178 degree 2 poles (-1.3898, 92.7811) (-1.3898, 92.4796) (-1.5519, 91.9578) (-1.6426, 91.786) knots 0 0 0 1 2 2 2
  line L242 (-1.6426, 91.786) -> (-2.2099, 91.786)
  line L243 (-2.2099, 91.786) -> (-2.2099, 91.8119)
  spline S179 degree 2 poles (-2.2099, 91.8119) (-2.158, 91.8767) (-2.0348, 92.0518) (-1.9668, 92.1976) knots 0 0 0 1 2 2 2
  spline S180 degree 2 poles (-1.9668, 92.1976) (-1.9052, 92.324) (-1.8144, 92.6352) (-1.8144, 92.8005) knots 0 0 0 1 2 2 2
  spline S181 degree 2 poles (-1.8144, 92.8005) (-1.8144, 92.9205) (-1.8695, 93.196) (-1.9149, 93.2608) knots 0 0 0 1 2 2 2
  spline S182 degree 2 poles (-1.9149, 93.2608) (-1.9765, 93.3548) (-2.1159, 93.4391) (-2.2585, 93.4391) knots 0 0 0 1 2 2 2
  spline S183 degree 2 poles (-2.2585, 93.4391) (-2.4368, 93.4391) (-2.6216, 93.2446) (-2.6831, 92.995) knots 0 0 0 1 2 2 2
  spline S184 degree 2 poles (-2.6831, 92.995) (-2.7058, 92.8978) (-2.7707, 92.5866) (-2.8063, 92.4537) knots 0 0 0 1 2 2 2
  spline S185 degree 2 poles (-2.8063, 92.4537) (-2.9068, 92.1101) (-3.3217, 91.7989) (-3.6167, 91.7989) knots 0 0 0 1 2 2 2
  spline S186 degree 2 poles (-3.6167, 91.7989) (-4.0251, 91.7989) (-4.534, 92.4116) (-4.534, 92.9172) knots 0 0 0 1 2 2 2
  spline S187 degree 2 poles (-4.534, 92.9172) (-4.534, 93.1668) (-4.4109, 93.6725) (-4.3169, 93.8443) knots 0 0 0 1 2 2 2
  line L244 (-4.3169, 93.8443) -> (-3.7755, 93.8443)
  line L245 (-3.7755, 93.8443) -> (-3.7755, 93.8184)
  spline S188 degree 2 poles (-3.7755, 93.8184) (-3.9311, 93.6239) (-4.1094, 93.1506) (-4.1094, 92.9075) knots 0 0 0 1 2 2 2
  spline S189 degree 2 poles (-4.1094, 92.9075) (-4.1094, 92.6579) (-3.8987, 92.3143) (-3.688, 92.3143) knots 0 0 0 1 2 2 2
  spline S190 degree 2 poles (-3.688, 92.3143) (-3.4968, 92.3143) (-3.312, 92.5185) (-3.2536, 92.7454) knots 0 0 0 1 2 2 2
  spline S191 degree 2 poles (-3.2536, 92.7454) (-3.2245, 92.8557) (-3.1661, 93.1344) (-3.1305, 93.2868) knots 0 0 0 1 2 2 2
  spline S192 degree 2 poles (-3.1305, 93.2868) (-3.0462, 93.6174) (-2.6605, 93.9545) (-2.3266, 93.9545) knots 0 0 0 1 2 2 2
  spline S193 degree 2 poles (-2.3266, 93.9545) (-2.1321, 93.9545) (-1.7885, 93.8022) (-1.6621, 93.6531) knots 0 0 0 1 2 2 2
  spline S194 degree 2 poles (-1.6621, 93.6531) (-1.5292, 93.4942) (-1.3898, 93.089) (-1.3898, 92.7811) knots 0 0 0 1 2 2 2
  line L246 (-1.4611, 95.209) -> (-1.4611, 94.5672)
  line L247 (-1.4611, 94.5672) -> (-2.2261, 94.5672)
  line L248 (-2.2261, 94.5672) -> (-2.2261, 95.209)
  line L249 (-2.2261, 95.209) -> (-1.4611, 95.209)
  line L250 (-5.6394, 96.6158) -> (-4.0835, 96.4991)
  line L251 (-4.0835, 96.4991) -> (-4.0835, 96.1458)
  line L252 (-4.0835, 96.1458) -> (-5.6394, 96.0291)
  line L253 (-5.6394, 96.0291) -> (-5.6394, 96.6158)
  line L254 (-5.6394, 97.6271) -> (-4.0835, 97.5104)
  line L255 (-4.0835, 97.5104) -> (-4.0835, 97.1571)
  line L256 (-4.0835, 97.1571) -> (-5.6394, 97.0404)
  line L257 (-5.6394, 97.0404) -> (-5.6394, 97.6271)
  point P0 (1.5, 80)
  dimension "d49" = 3.2481
  dimension "d50" = 101.462
  dimension "d51" = 3.8913
  dimension "d52" = 22.3274
  constraints: 1 vertical, 2 other
  measures "d49" distance between parallel lines of L2 L0
  measures "d50" distance between parallel lines of L3 L1
  measures "d51" distance from line of point (1.5, 80) L2
  measures "d52" distance from line of point (1.5, 80) L1
emboss "Emboss1" sketch "Sketch11" operation cut depth 1 direction (1, 0, 0)
extrude "Extrusion7" cut sketch "Sketch9" against normal blind 20
body "Solid1"
